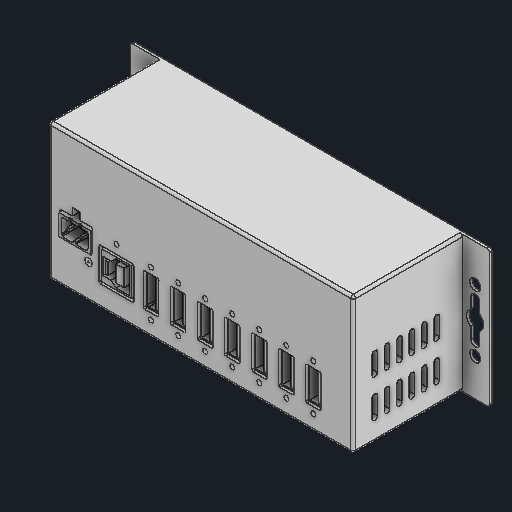
# Autodesk Inventor part: StarTech7PortUSB3Hub
Saved by Autodesk Inventor 2025.2 (Build 292293000, 293)
## iProperties
Created: 2025-10-31
Part Number: StarTech7PortUSB3Hub
Material: Generic
Document SubType Name: Modeling
Designer: valer
Density: 1 g/cm^3
Appearance: Default
Author: valer
Autodesk Inventor part; units mm, degrees
ref_plane "YZ Plane" through (0, 0, 0) normal (1, 0, 0) x (0, 1, 0)
ref_plane "XZ Plane" through (0, 0, 0) normal (0, 1, 0) x (-1, 0, 0)
ref_plane "XY Plane" through (0, 0, 0) normal (0, 0, 1) x (1, 0, 0)
sketch "Base" plane through (0, 0, 0) normal (0, 0, 1) x (1, 0, 0)
  line L0 (-72.5, -27.5) -> (72.5, -27.5)
  line L1 (72.5, -27.5) -> (72.5, 27.5)
  line L2 (72.5, 27.5) -> (-72.5, 27.5)
  line L3 (-72.5, 27.5) -> (-72.5, -27.5)
  line L4 (-72.5, -27.5) -> (72.5, 27.5) construction
  line L5 (72.5, -27.5) -> (-72.5, 27.5) construction
  line L6 (-66.75, 27.5) -> (-66.75, -27.5) construction
  line L7 (-101.5, 0) -> (101.5, 0) construction
  line L8 (0, -38.5) -> (0, 38.5) construction
  line L9 (66.75, 27.5) -> (66.75, -27.5) construction
  circle A0 centre (-66.75, 12.5) radius 2.25
  circle A1 centre (-66.75, -12.5) radius 2.25
  circle A2 centre (66.75, 12.5) radius 2.25
  circle A3 centre (66.75, -12.5) radius 2.25
  circle A4 centre (-66.75, 0) radius 3.5
  circle A5 centre (66.75, 0) radius 3.5
  circle A6 centre (-66.75, 7.5) radius 1.75
  circle A7 centre (-66.75, -7.5) radius 1.75
  line L10 (-68.5, 7.5) -> (-68.5, -7.5)
  line L11 (-65, 7.5) -> (-65, -7.5)
  circle A8 centre (66.75, 7.5) radius 1.75
  circle A9 centre (66.75, -7.5) radius 1.75
  line L12 (68.5, 7.5) -> (68.5, -7.5)
  line L13 (65, 7.5) -> (65, -7.5)
  line L14 (-70.25, 3.5) -> (-63.25, 3.5)
  line L15 (-63.25, 3.5) -> (-63.25, -3.5)
  line L16 (-63.25, -3.5) -> (-70.25, -3.5)
  line L17 (-70.25, -3.5) -> (-70.25, 3.5)
  point P0 (0, 0)
  point P1 (-65, -3.0311)
  point P2 (-68.5, -3.0311)
  point P3 (-68.5, 3.0311)
  point P4 (-65, 3.0311)
  point P5 (65, -3.0311)
  point P6 (65, 3.0311)
  point P7 (68.5, 3.0311)
  point P8 (68.5, -3.0311)
  dimension "d15" = 1
  dimension "d0" = 145
  dimension "d1" = 55
  dimension "d2" = 133.5
  dimension "d3" = 4.5
  dimension "d4" = 15
  dimension "d5" = 7
  dimension "d6" = 3.5
  dimension "d7" = 20
  dimension "d63" = 2.25
  constraints: 32 end point, 13 symmetric about line, 10 centre point, 8 point on circle, 8 tangent, 5 point on line, 4 parallel, 3 midpoint, 3 perpendicular, 2 horizontal, 7 other
  measures "d0" distance of L1.end L2.end
  measures "d1" distance of L0.end L1.end
  measures "d2" distance between parallel lines of L9 L6
  measures "d3" diameter of A0
  measures "d4" distance from line of L2 A0.centre
  measures "d5" diameter of A4
  measures "d6" diameter of A6
  measures "d7" distance of A1.centre A6.centre
  measures "d63" distance between parallel lines of L3 L17
extrude "BaseFeature" add sketch "Base" along normal blind 1 contours L3 L2 L1 L0 | L15 L16 L11 A4 | A4 L11 L14 L15 | A4 L17 L14 L10 | L10 L16 L17 A4
fillet "BaseFilletsFeature" radius 1 4 edges at (-72.5, -27.5, 0.5) (-72.5, 27.5, 0.5) (72.5, -27.5, 0.5) (72.5, 27.5, 0.5)
sketch "Sketch2" plane through (0, 0, 1) normal (0, 0, 1) x (1, 0, 0)
  line L0 (71.5, 27.5) -> (-71.5, 27.5) projected
  line L1 (-71.5, -27.5) -> (71.5, -27.5) projected
  line L2 (-61.5, 27.5) -> (61.5, 27.5)
  line L3 (61.5, 27.5) -> (61.5, -27.5)
  line L4 (61.5, -27.5) -> (-61.5, -27.5)
  line L5 (-61.5, -27.5) -> (-61.5, 27.5)
  line L6 (-72.5, 26.5) -> (-72.5, -26.5) projected
  line L7 (72.5, -26.5) -> (72.5, 26.5) projected
  point P0 (0, 0)
  point P1 (-61.5, -27.5)
  point P2 (61.5, 27.5)
  dimension "d11" = 11
  dimension "d12" = 11
  constraints: 8 end point, 2 parallel, 2 point on line, 1 horizontal, 1 perpendicular
  measures "d11" distance between parallel lines of L6 L5
  measures "d12" distance between parallel lines of L7 L3
extrude "BodyFeature" add sketch "Sketch2" along normal blind 44
fillet "BodyFilletsFeature" radius 1 4 edges at (-61.5, -27.5, 23) (-61.5, 27.5, 23) (61.5, -27.5, 23) (61.5, 27.5, 23)
sketch "Sketch3" plane through (0, 0, 45) normal (0, 0, 1) x (1, 0, 0)
  line L0 (-41.05, -1.85) -> (48.52, -1.85) construction
  line L1 (48.52, -1.85) -> (48.52, -22.35) construction
  line L2 (48.52, -22.35) -> (-41.05, -22.35) construction
  line L3 (-41.05, -22.35) -> (-41.05, -1.85) construction
  arc A0 (65, 3.0311) -> (65, -3.0311) centre (66.75, 0) ccw projected
  line L4 (48.52, -2.85) -> (-41.05, -2.85) construction
  line L5 (48.52, -12.1) -> (-41.05, -12.1) construction
  circle A1 centre (45.42, -2.85) radius 1
  line L6 (42.32, -5.35) -> (48.52, -5.35)
  line L7 (48.52, -5.35) -> (48.52, -18.85)
  line L8 (48.52, -18.85) -> (42.32, -18.85)
  line L9 (42.32, -18.85) -> (42.32, -5.35)
  line L10 (45.42, -2.85) -> (45.42, -12.1) construction
  circle A2 centre (45.42, -21.35) radius 1
  line L11 (61.5, -26.5) -> (61.5, 26.5) construction
  line L12 (31.4, -5.35) -> (37.6, -5.35)
  line L13 (31.4, -18.85) -> (31.4, -5.35)
  line L14 (37.6, -18.85) -> (31.4, -18.85)
  line L15 (37.6, -5.35) -> (37.6, -18.85)
  circle A3 centre (34.5, -2.85) radius 1
  circle A4 centre (34.5, -21.35) radius 1
  line L16 (20.48, -5.35) -> (26.68, -5.35)
  line L17 (20.48, -18.85) -> (20.48, -5.35)
  line L18 (26.68, -18.85) -> (20.48, -18.85)
  line L19 (26.68, -5.35) -> (26.68, -18.85)
  circle A5 centre (23.58, -2.85) radius 1
  circle A6 centre (23.58, -21.35) radius 1
  line L20 (9.56, -5.35) -> (15.76, -5.35)
  line L21 (9.56, -18.85) -> (9.56, -5.35)
  line L22 (15.76, -18.85) -> (9.56, -18.85)
  line L23 (15.76, -5.35) -> (15.76, -18.85)
  circle A7 centre (12.66, -2.85) radius 1
  circle A8 centre (12.66, -21.35) radius 1
  line L24 (-1.36, -5.35) -> (4.84, -5.35)
  line L25 (-1.36, -18.85) -> (-1.36, -5.35)
  line L26 (4.84, -18.85) -> (-1.36, -18.85)
  line L27 (4.84, -5.35) -> (4.84, -18.85)
  circle A9 centre (1.74, -2.85) radius 1
  circle A10 centre (1.74, -21.35) radius 1
  line L28 (-12.28, -5.35) -> (-6.08, -5.35)
  line L29 (-12.28, -18.85) -> (-12.28, -5.35)
  line L30 (-6.08, -18.85) -> (-12.28, -18.85)
  line L31 (-6.08, -5.35) -> (-6.08, -18.85)
  circle A11 centre (-9.18, -2.85) radius 1
  circle A12 centre (-9.18, -21.35) radius 1
  line L32 (-23.2, -5.35) -> (-17, -5.35)
  line L33 (-23.2, -18.85) -> (-23.2, -5.35)
  line L34 (-17, -18.85) -> (-23.2, -18.85)
  line L35 (-17, -5.35) -> (-17, -18.85)
  circle A13 centre (-20.1, -2.85) radius 1
  circle A14 centre (-20.1, -21.35) radius 1
  line L36 (-27.05, -5.35) -> (-41.05, -5.35)
  line L37 (-41.05, -5.35) -> (-41.05, -18.85)
  line L38 (-41.05, -18.85) -> (-27.05, -18.85)
  line L39 (-27.05, -18.85) -> (-27.05, -5.35)
  line L40 (-34.05, -2.85) -> (-34.05, -22.35) construction
  line L41 (-56.85, -0.85) -> (-43.85, -0.85)
  line L42 (-43.85, -0.85) -> (-43.85, -10.25)
  line L43 (-43.85, -10.25) -> (-56.85, -10.25)
  line L44 (-56.85, -10.25) -> (-56.85, -0.85)
  line L45 (-61.5, 26.5) -> (-61.5, -26.5) construction
  circle A15 centre (-34.05, -1.85) radius 1
  circle A16 centre (-34.05, -22.35) radius 1
  circle A17 centre (-45.35, -13.6) radius 1.5
  line L46 (-43.85, -10.25) -> (-43.85, -13.6) construction
  line L47 (-41.05, -12.1) -> (-45.35, -12.1) construction
  line L48 (-51.85, -0.85) -> (-48.85, -0.85)
  line L49 (-48.85, -0.85) -> (-48.85, 2.15)
  line L50 (-48.85, 2.15) -> (-51.85, 2.15)
  line L51 (-51.85, 2.15) -> (-51.85, -0.85)
  line L52 (-50.35, -10.25) -> (-50.35, -0.85) construction
  point P0 (0, 0)
  point P1 (42.32, -12.1)
  point P2 (45.42, -5.35)
  point P3 (34.5, -5.35)
  point P4 (31.4, -12.1)
  point P5 (23.58, -5.35)
  point P6 (20.48, -12.1)
  point P7 (12.66, -5.35)
  point P8 (9.56, -12.1)
  point P9 (1.74, -5.35)
  point P10 (-1.36, -12.1)
  point P11 (-9.18, -5.35)
  point P12 (-12.28, -12.1)
  point P13 (-20.1, -5.35)
  point P14 (-23.2, -12.1)
  point P15 (-34.05, -5.35)
  point P16 (-27.05, -12.1)
  point P17 (-50.35, -0.85)
  dimension "d16" = 12.1
  dimension "d17" = 2
  dimension "d18" = 13.5
  dimension "d19" = 6.2
  dimension "d20" = 18.5
  dimension "d21" = 12.98
  dimension "d24" = 10.92
  dimension "d29" = 14
  dimension "d30" = 13.95
  dimension "d31" = 16.3
  dimension "d32" = 9.4
  dimension "d33" = 11.15
  dimension "d34" = 1
  dimension "d35" = 13
  dimension "d36" = 3
  dimension "d64" = 3
  constraints: 102 end point, 17 centre point, 13 point on line, 10 midpoint, 10 parallel, 9 perpendicular, 6 horizontal, 4 collinear, 3 tangent, 2 equal length, 2 equal radius, 2 point on circle, 1 coincident, 1 symmetric about line, 85 other
  measures "d16" vertical distance of A0.centre L5.start
  measures "d17" diameter of A1
  measures "d18" distance of L6.end L7.end
  measures "d19" distance between parallel lines of L9 L7
  measures "d20" distance from line of A2.centre L4
  measures "d21" distance between parallel lines of L11 L1
  measures "d24" distance of L6.start L12.start
  measures "d29" distance of L37.end L38.end
  measures "d30" distance from line of A14.centre L40
  measures "d31" distance from line of L52.start L40
  measures "d32" distance of L41.end L42.end
  measures "d33" distance from line of L45 L52.start
  measures "d34" distance between parallel lines of L0 L41
  measures "d35" distance of L42.end L43.end
  measures "d36" diameter of A17
  measures "d64" distance of L49.end L50.end
extrude "PortsFeature" cut sketch "Sketch3" against normal blind 6 contours A1 | L6 L7 L8 L9 | A2 | L12 L15 L14 L13 | A3 | A4 | L16 L19 L18 L17 | A5 | A6 | L20 L23 L22 L21 | A7 | A8 | L24 L27 L26 L25 | A9 | A10 | L28 L31 L30 L29 | A11 | A12 | L32 L35 L34 L33 | A13 | A14 | L39 L38 L37 L36 | L41 L42 L43 L44 | L51 L50 L49 L41 | A15 | A17
fillet "PortFilletsFeature" radius 0.5 36 edges at (48.52, -5.35, 42) (42.32, -5.35, 42) (42.32, -18.85, 42) (48.52, -18.85, 42) (37.6, -5.35, 42) (31.4, -5.35, 42) (31.4, -18.85, 42) (37.6, -18.85, 42) (26.68, -5.35, 42) (20.48, -5.35, 42) (20.48, -18.85, 42) (26.68, -18.85, 42) (15.76, -5.35, 42) (9.56, -5.35, 42) (9.56, -18.85, 42) (15.76, -18.85, 42) (4.84, -5.35, 42) (-1.36, -5.35, 42) (-1.36, -18.85, 42) (4.84, -18.85, 42) (-6.08, -5.35, 42) (-12.28, -5.35, 42) (-12.28, -18.85, 42) (-6.08, -18.85, 42) (-17, -5.35, 42) (-23.2, -5.35, 42) (-23.2, -18.85, 42) (-17, -18.85, 42) (-27.05, -5.35, 42) (-41.05, -5.35, 42) (-41.05, -18.85, 42) (-27.05, -18.85, 42) (-43.85, -0.85, 42) (-56.85, -0.85, 42) (-56.85, -10.25, 42) (-43.85, -10.25, 42)
fillet "OutsideFilletsFeature" radius 1 8 edges at (-61.2071, 27.2071, 45) (-61.5, 0, 45) (-61.2071, -27.2071, 45) (0, -27.5, 45) (61.2071, -27.2071, 45) (61.5, 0, 45) (61.2071, 27.2071, 45) (0, 27.5, 45)
sketch "Vents" plane through (61.5, -26.5, 1) normal (1, 0, 0) x (0, 0, -1)
  line L0 (-44, 7.65) -> (-38, 7.65) construction
  line L1 (-35.35, 7.65) -> (0, 7.65) construction
  line L2 (0, 7.65) -> (0, 15.65) construction
  line L3 (0, 15.65) -> (-35.35, 15.65) construction
  line L4 (-35.35, 15.65) -> (-35.35, 7.65) construction
  line L5 (-43, -1) -> (0, -1) projected
  line L6 (-44, 53) -> (-44, 0) projected
  line L7 (-35.35, 22.85) -> (-35.35, 14.85) construction
  line L8 (-35.35, 14.85) -> (0, 14.85) construction
  line L9 (0, 22.85) -> (-35.35, 22.85) construction
  line L10 (0, 14.85) -> (0, 22.85) construction
  line L11 (-35.35, 30.05) -> (-35.35, 22.05) construction
  line L12 (-35.35, 22.05) -> (0, 22.05) construction
  line L13 (0, 30.05) -> (-35.35, 30.05) construction
  line L14 (0, 22.05) -> (0, 30.05) construction
  line L15 (-35.35, 7.65) -> (-35.35, 14.85) construction
  line L16 (-34.25, 7.65) -> (-34.25, 14.85)
  line L17 (-36.45, 14.85) -> (-36.45, 7.65)
  arc A0 (-36.45, 7.65) -> (-34.25, 7.65) centre (-35.35, 7.65) ccw
  arc A1 (-34.25, 14.85) -> (-36.45, 14.85) centre (-35.35, 14.85) ccw
  line L18 (0, 0) -> (0, 53) projected
  line L19 (-35.35, 18.85) -> (0, 18.85) construction
  line L20 (-34.25, 30.05) -> (-34.25, 22.85)
  line L21 (-36.45, 22.85) -> (-36.45, 30.05)
  arc A2 (-34.25, 30.05) -> (-36.45, 30.05) centre (-35.35, 30.05) ccw
  arc A3 (-36.45, 22.85) -> (-34.25, 22.85) centre (-35.35, 22.85) ccw
  arc A4 (-31.45, 7.65) -> (-29.25, 7.65) centre (-30.35, 7.65) ccw
  line L22 (-31.45, 14.85) -> (-31.45, 7.65)
  line L23 (-29.25, 7.65) -> (-29.25, 14.85)
  arc A5 (-29.25, 14.85) -> (-31.45, 14.85) centre (-30.35, 14.85) ccw
  arc A6 (-31.45, 22.85) -> (-29.25, 22.85) centre (-30.35, 22.85) ccw
  line L24 (-31.45, 22.85) -> (-31.45, 30.05)
  line L25 (-29.25, 30.05) -> (-29.25, 22.85)
  arc A7 (-29.25, 30.05) -> (-31.45, 30.05) centre (-30.35, 30.05) ccw
  arc A8 (-26.45, 7.65) -> (-24.25, 7.65) centre (-25.35, 7.65) ccw
  line L26 (-26.45, 14.85) -> (-26.45, 7.65)
  line L27 (-24.25, 7.65) -> (-24.25, 14.85)
  arc A9 (-24.25, 14.85) -> (-26.45, 14.85) centre (-25.35, 14.85) ccw
  arc A10 (-26.45, 22.85) -> (-24.25, 22.85) centre (-25.35, 22.85) ccw
  line L28 (-26.45, 22.85) -> (-26.45, 30.05)
  line L29 (-24.25, 30.05) -> (-24.25, 22.85)
  arc A11 (-24.25, 30.05) -> (-26.45, 30.05) centre (-25.35, 30.05) ccw
  arc A12 (-21.45, 7.65) -> (-19.25, 7.65) centre (-20.35, 7.65) ccw
  line L30 (-21.45, 14.85) -> (-21.45, 7.65)
  line L31 (-19.25, 7.65) -> (-19.25, 14.85)
  arc A13 (-19.25, 14.85) -> (-21.45, 14.85) centre (-20.35, 14.85) ccw
  arc A14 (-21.45, 22.85) -> (-19.25, 22.85) centre (-20.35, 22.85) ccw
  line L32 (-21.45, 22.85) -> (-21.45, 30.05)
  line L33 (-19.25, 30.05) -> (-19.25, 22.85)
  arc A15 (-19.25, 30.05) -> (-21.45, 30.05) centre (-20.35, 30.05) ccw
  arc A16 (-16.45, 7.65) -> (-14.25, 7.65) centre (-15.35, 7.65) ccw
  line L34 (-16.45, 14.85) -> (-16.45, 7.65)
  line L35 (-14.25, 7.65) -> (-14.25, 14.85)
  arc A17 (-14.25, 14.85) -> (-16.45, 14.85) centre (-15.35, 14.85) ccw
  arc A18 (-16.45, 22.85) -> (-14.25, 22.85) centre (-15.35, 22.85) ccw
  line L36 (-16.45, 22.85) -> (-16.45, 30.05)
  line L37 (-14.25, 30.05) -> (-14.25, 22.85)
  arc A19 (-14.25, 30.05) -> (-16.45, 30.05) centre (-15.35, 30.05) ccw
  arc A20 (-11.45, 7.65) -> (-9.25, 7.65) centre (-10.35, 7.65) ccw
  line L38 (-11.45, 14.85) -> (-11.45, 7.65)
  line L39 (-9.25, 7.65) -> (-9.25, 14.85)
  arc A21 (-9.25, 14.85) -> (-11.45, 14.85) centre (-10.35, 14.85) ccw
  arc A22 (-11.45, 22.85) -> (-9.25, 22.85) centre (-10.35, 22.85) ccw
  line L40 (-11.45, 22.85) -> (-11.45, 30.05)
  line L41 (-9.25, 30.05) -> (-9.25, 22.85)
  arc A23 (-9.25, 30.05) -> (-11.45, 30.05) centre (-10.35, 30.05) ccw
  point P0 (1, 26.5)
  point P1 (-35.35, 11.25)
  dimension "d41" = 8.65
  dimension "d42" = 8.65
  dimension "d46" = 7.2
  dimension "d51" = 1.1
  dimension "d54" = 5
  dimension "d59" = 7.2
  dimension "d60" = 8
  constraints: 78 end point, 48 point on circle, 24 centre point, 5 symmetric about line, 4 tangent, 3 collinear, 3 parallel, 2 horizontal, 2 midpoint, 2 perpendicular, 2 point on line, 1 vertical, 117 other
  measures "d41" distance between parallel lines of L5 L0
  measures "d42" distance between parallel lines of L6 L4
  measures "d46" distance of L3.end L7.start
  measures "d51" radius of A1
  measures "d54" distance of L1.start A4.centre
  measures "d59" distance between parallel lines of L0 L8
  measures "d60" distance between parallel lines of L9 L8
extrude "VentsFeature" cut sketch "Vents" against normal blind 20
sketch "Sketch5" plane through (-45.35, -13.6, 39) normal (0, 0, 1) x (1, 0, 0)
  circle A0 centre (0, 0) radius 1.5 projected
  circle A1 centre (0, 0) radius 1.3
  point P0 (45.35, 13.6)
  dimension "d65" = 0.2
  constraints: 1 centre point
  measures "d65" radial gap between concentric circles of A0 A1
extrude "Extrusion5" add sketch "Sketch5" along normal blind 6 contours A1
fillet "Fillet5" radius 1 1 edges at (-46.65, -13.6, 45)
sketch "Sketch6" plane through (0, 0, 39) normal (0, 0, 1) x (1, 0, 0)
  line L0 (-56.85, -1.85) -> (-43.85, -1.85)
  line L1 (-43.85, -1.85) -> (-43.85, -10.25)
  line L2 (-43.85, -10.25) -> (-56.85, -10.25)
  line L3 (-56.85, -10.25) -> (-56.85, -1.85)
  line L4 (-48.85, -0.85) -> (-44.35, -0.85) projected
  line L5 (-43.85, -1.35) -> (-43.85, -9.75) projected
  line L6 (-44.35, -10.25) -> (-56.35, -10.25) projected
  line L7 (-56.85, -9.75) -> (-56.85, -1.35) projected
  line L8 (-44.85, -2.85) -> (-55.85, -2.85)
  line L9 (-55.85, -2.85) -> (-55.85, -9.25)
  line L10 (-55.85, -9.25) -> (-44.85, -9.25) construction
  line L11 (-44.85, -9.25) -> (-44.85, -2.85)
  line L12 (-50.35, -2.85) -> (-50.35, -9.25) construction
  arc A0 (-55.85, -9.25) -> (-50.35, -9.25) centre (-53.1, 0.3644) ccw
  arc A1 (-50.35, -9.25) -> (-44.85, -9.25) centre (-47.6, 0.3644) ccw
  line L13 (-55.85, -2.85) -> (-50.35, -9.25) construction
  line L14 (-50.35, -9.25) -> (-44.85, -2.85) construction
  line L15 (-53.6, -5.55) -> (-52.6, -5.55)
  line L16 (-52.6, -5.55) -> (-52.6, -6.55)
  line L17 (-52.6, -6.55) -> (-53.6, -6.55)
  line L18 (-53.6, -6.55) -> (-53.6, -5.55)
  line L19 (-53.6, -5.55) -> (-52.6, -6.55) construction
  line L20 (-52.6, -5.55) -> (-53.6, -6.55) construction
  line L21 (-47.1, -5.55) -> (-48.1, -5.55)
  line L22 (-48.1, -5.55) -> (-48.1, -6.55)
  line L23 (-48.1, -6.55) -> (-47.1, -6.55)
  line L24 (-47.1, -6.55) -> (-47.1, -5.55)
  point P0 (0, 0)
  point P1 (-53.1, -6.05)
  dimension "d69" = 1
  dimension "d70" = 1
  dimension "d71" = 10
  dimension "d72" = 1
  constraints: 42 end point, 6 parallel, 5 midpoint, 4 perpendicular, 4 point on circle, 4 symmetric about line, 3 collinear, 2 centre point, 2 horizontal, 1 equal radius, 3 other
  measures "d69" distance between parallel lines of L0 L4
  measures "d70" distance between parallel lines of L0 L8
  measures "d71" radius of A0
  measures "d72" distance of L15.end L16.end
extrude "Extrusion6" add sketch "Sketch6" along normal blind 6.5
sketch "Sketch7" plane through (0, 0, 45.5) normal (0, 0, 1) x (1, 0, 0)
  line L0 (-43.85, -1.85) -> (-56.85, -1.85) projected
  line L1 (-44.85, -2.85) -> (-44.85, -9.25) projected
  arc A0 (-50.35, -9.25) -> (-44.85, -9.25) centre (-47.6, 0.3644) ccw projected
  arc A1 (-55.85, -9.25) -> (-50.35, -9.25) centre (-53.1, 0.3644) ccw projected
  line L2 (-55.85, -9.25) -> (-55.85, -2.85) projected
  line L3 (-55.85, -2.85) -> (-44.85, -2.85) projected
  line L4 (-56.35, -9.75) -> (-55.35, -9.75)
  line L5 (-55.35, -9.75) -> (-55.35, -8.75)
  line L6 (-55.35, -8.75) -> (-56.35, -8.75)
  line L7 (-56.35, -8.75) -> (-56.35, -9.75)
  line L8 (-56.35, -9.75) -> (-55.35, -8.75) construction
  line L9 (-55.35, -9.75) -> (-56.35, -8.75) construction
  line L10 (-55.85, -2.85) -> (-55.85, -9.25) projected
  line L11 (-55.85, -6.05) -> (-44.85, -6.05) construction
  line L12 (-50.35, -2.85) -> (-50.35, -9.25) construction
  line L13 (-44.35, -9.75) -> (-45.35, -9.75)
  line L14 (-45.35, -9.75) -> (-45.35, -8.75)
  line L15 (-45.35, -8.75) -> (-44.35, -8.75)
  line L16 (-44.35, -8.75) -> (-44.35, -9.75)
  line L17 (-56.35, -2.35) -> (-55.35, -2.35)
  line L18 (-55.35, -2.35) -> (-55.35, -3.35)
  line L19 (-55.35, -3.35) -> (-56.35, -3.35)
  line L20 (-56.35, -3.35) -> (-56.35, -2.35)
  line L21 (-45.35, -2.35) -> (-45.35, -3.35)
  line L22 (-45.35, -3.35) -> (-44.35, -3.35)
  line L23 (-44.35, -3.35) -> (-44.35, -2.35)
  line L24 (-44.35, -2.35) -> (-45.35, -2.35)
  line L25 (-50.85, -9.75) -> (-49.85, -9.75)
  line L26 (-49.85, -9.75) -> (-49.85, -8.75)
  line L27 (-49.85, -8.75) -> (-50.85, -8.75)
  line L28 (-50.85, -8.75) -> (-50.85, -9.75)
  line L29 (-50.85, -9.75) -> (-49.85, -8.75) construction
  line L30 (-49.85, -9.75) -> (-50.85, -8.75) construction
  line L31 (-55.85, -8.75) -> (-55.35, -8.75)
  line L32 (-55.35, -8.75) -> (-55.35, -9.3791)
  line L33 (-56.85, -1.85) -> (-56.85, -10.25) projected
  line L34 (-56.85, -10.25) -> (-43.85, -10.25) projected
  line L35 (-43.85, -10.25) -> (-43.85, -1.85) projected
  point P0 (0, 0)
  point P1 (-50.85, -9.3791)
  point P2 (-49.85, -9.3791)
  point P3 (-44.85, -8.75)
  point P4 (-45.35, -9.3791)
  dimension "d75" = 1
  constraints: 56 end point, 12 symmetric about line, 8 midpoint, 4 parallel, 3 equal length, 2 horizontal, 2 perpendicular, 2 point on line, 1 collinear, 1 point on circle, 1 vertical
  measures "d75" distance of L6.end L5.end
extrude "Extrusion7" add sketch "Sketch7" against normal up to surface (6.5 mm away) contours L3 L21 L24 L23 L22 L1 | L1 L22 L21 L3 | L1 A0 L14 L15 | L18 L19 L2 L3 | L3 L2 L19 L20 L17 L18 | A0 A1 L28 L27 L26 | L6 L5 A1 L2
sketch "Sketch8" plane through (0, 0, 45.5) normal (0, 0, 1) x (1, 0, 0)
  line L0 (-50.85, -8.75) -> (-49.85, -8.75) construction
  line L1 (-50.35, -8.75) -> (-50.35, -1.85) construction
  line L2 (-43.85, -1.85) -> (-56.85, -1.85) construction
  line L3 (-55.35, -2.85) -> (-45.35, -2.85) projected
  line L4 (-52.85, -1.85) -> (-51.85, -1.85)
  line L5 (-51.85, -1.85) -> (-51.85, -2.85)
  line L6 (-51.85, -2.85) -> (-52.85, -2.85)
  line L7 (-52.85, -2.85) -> (-52.85, -1.85)
  line L8 (-51.85, -0.85) -> (-51.85, 2.15) projected
  line L9 (-47.85, -1.85) -> (-48.85, -1.85)
  line L10 (-48.85, -1.85) -> (-48.85, -2.85)
  line L11 (-48.85, -2.85) -> (-47.85, -2.85)
  line L12 (-47.85, -2.85) -> (-47.85, -1.85)
  point P0 (0, 0)
  dimension "d78" = 1
  constraints: 18 end point, 4 symmetric about line, 2 midpoint, 2 parallel, 2 point on line, 1 collinear, 1 horizontal, 1 perpendicular
  measures "d78" distance between parallel lines of L5 L7
extrude "Extrusion8" cut sketch "Sketch8" against normal blind 0.5
sketch "Sketch9" plane through (0, 0, 39) normal (0, 0, 1) x (1, 0, 0)
  line L0 (-28.05, -6.35) -> (-40.05, -6.35)
  line L1 (-40.05, -6.35) -> (-40.05, -17.85)
  line L2 (-40.05, -17.85) -> (-28.05, -17.85)
  line L3 (-28.05, -17.85) -> (-28.05, -6.35)
  line L4 (-40.05, -12.1) -> (-28.05, -12.1) construction
  line L5 (-39.55, -12.1) -> (-39.55, -8.7282)
  line L6 (-39.55, -8.7282) -> (-36.25, -8.7282)
  line L7 (-36.25, -8.7282) -> (-34.25, -7.05)
  line L8 (-34.25, -7.05) -> (-28.75, -7.05)
  line L9 (-28.75, -7.05) -> (-28.75, -12.1)
  line L10 (-40.55, -5.35) -> (-27.55, -5.35) projected
  line L11 (-27.05, -5.85) -> (-27.05, -18.35) projected
  line L12 (-41.05, -18.35) -> (-41.05, -5.85) projected
  line L13 (-27.55, -18.85) -> (-40.55, -18.85) projected
  line L14 (-39.55, -12.1) -> (-39.55, -15.4718)
  line L15 (-39.55, -15.4718) -> (-36.25, -15.4718)
  line L16 (-36.25, -15.4718) -> (-34.25, -17.15)
  line L17 (-34.25, -17.15) -> (-28.75, -17.15)
  line L18 (-28.75, -17.15) -> (-28.75, -12.1)
  line L19 (-34.25, -15.45) -> (-31.05, -15.45)
  line L20 (-31.05, -15.45) -> (-31.05, -8.75)
  line L21 (-31.05, -8.75) -> (-34.25, -8.75)
  line L22 (-34.25, -8.75) -> (-34.25, -15.45)
  line L23 (-34.25, -15.45) -> (-31.05, -8.75) construction
  line L24 (-31.05, -15.45) -> (-34.25, -8.75) construction
  line L25 (-34.25, -7.05) -> (-34.25, -8.75) construction
  line L26 (-38.55, -14.4718) -> (-38.55, -9.7282)
  line L27 (-38.55, -9.7282) -> (-37.55, -9.7282)
  line L28 (-37.55, -9.7282) -> (-37.55, -14.4718)
  line L29 (-37.55, -14.4718) -> (-38.55, -14.4718)
  line L30 (-38.55, -14.4718) -> (-37.55, -9.7282) construction
  line L31 (-38.55, -9.7282) -> (-37.55, -14.4718) construction
  point P0 (0, 0)
  point P1 (-32.65, -12.1)
  point P2 (-38.05, -12.1)
  dimension "d81" = 1
  dimension "d82" = 1
  dimension "d83" = 1
  dimension "d84" = 0.5
  dimension "d85" = 0.7
  dimension "d86" = 0.7
  dimension "d87" = 140
  dimension "d88" = 3.3
  dimension "d89" = 5.5
  dimension "d90" = 1
  dimension "d91" = 2.3
  dimension "d92" = 1.7
  dimension "d95" = 1
  dimension "d96" = 1
  dimension "d97" = 1
  constraints: 56 end point, 7 parallel, 7 perpendicular, 6 midpoint, 4 point on line, 4 symmetric about line, 2 horizontal, 1 vertical
  measures "d81" distance between parallel lines of L10 L0
  measures "d82" distance between parallel lines of L11 L3
  measures "d83" distance between parallel lines of L12 L1
  measures "d84" distance between parallel lines of L1 L5
  measures "d85" distance between parallel lines of L0 L8
  measures "d86" distance between parallel lines of L3 L9
  measures "d87" angle of L6 L7
  measures "d88" distance of L5.end L6.end
  measures "d89" distance of L7.end L8.end
  measures "d90" distance between parallel lines of L13 L2
  measures "d91" distance between parallel lines of L9 L20
  measures "d92" distance between parallel lines of L8 L21
  measures "d95" distance between parallel lines of L6 L27
  measures "d96" distance between parallel lines of L5 L26
  measures "d97" distance of L26.end L27.end
extrude "Extrusion9" add sketch "Sketch9" along normal up to surface (6 mm away)
sketch "Sketch10" plane through (0, 0, 39) normal (0, 0, 1) x (1, 0, 0)
  line L0 (-23.2, -18.35) -> (-23.2, -5.85) construction
  line L1 (-23.2, -12.1) -> (-17, -12.1) construction
  line L2 (-17, -5.85) -> (-17, -18.35) construction
  line L3 (-23.0536, -12.1) -> (-23.0536, -5.4964)
  line L4 (-23.0536, -5.4964) -> (-17.1464, -5.4964)
  line L5 (-17.1464, -5.4964) -> (-17.1464, -12.1)
  arc A0 (-22.7, -5.35) -> (-23.2, -5.85) centre (-22.7, -5.85) ccw projected
  arc A1 (-17, -5.85) -> (-17.5, -5.35) centre (-17.5, -5.85) ccw projected
  line L6 (-17.6464, -12.1) -> (-17.6464, -5.9964)
  line L7 (-17.6464, -5.9964) -> (-22.5536, -5.9964)
  line L8 (-22.5536, -5.9964) -> (-22.5536, -12.1)
  line L9 (-23.0536, -12.1) -> (-23.0536, -18.7036)
  line L10 (-23.0536, -18.7036) -> (-17.1464, -18.7036)
  line L11 (-17.1464, -18.7036) -> (-17.1464, -12.1)
  line L12 (-17.6464, -12.1) -> (-17.6464, -18.2036)
  line L13 (-17.6464, -18.2036) -> (-22.5536, -18.2036)
  line L14 (-22.5536, -18.2036) -> (-22.5536, -12.1)
  point P0 (0, 0)
  dimension "d101" = 0.5
  constraints: 26 end point, 4 symmetric about line, 3 perpendicular, 2 midpoint, 2 point on circle, 2 point on line, 1 vertical, 2 other
  measures "d101" distance between parallel lines of L4 L7
extrude "Extrusion10" add sketch "Sketch10" along normal blind 5 separate body
chamfer "Chamfer2" distance 0.5 angle 45 8 edges at (-23.0536, -5.4964, 41.5) (-17.1464, -5.4964, 41.5) (-23.0536, -18.7036, 41.5) (-17.1464, -18.7036, 41.5) (-22.5536, -5.9964, 41.5) (-17.6464, -5.9964, 41.5) (-22.5536, -18.2036, 41.5) (-17.6464, -18.2036, 41.5)
sketch "Sketch11" plane through (0, 0, 39) normal (0, 0, 1) x (1, 0, 0)
  line L0 (-18.1464, -6.4964) -> (-19.1464, -6.4964)
  line L1 (-19.1464, -6.4964) -> (-19.1464, -17.7036)
  line L2 (-19.1464, -17.7036) -> (-18.1464, -17.7036)
  line L3 (-18.1464, -17.7036) -> (-18.1464, -6.4964)
  line L4 (-22.0536, -5.9964) -> (-18.1464, -5.9964) projected
  line L5 (-18.1464, -6.4964) -> (-18.1464, -5.9964) construction
  line L6 (-22.0536, -5.9964) -> (-18.1464, -5.9964) projected
  line L7 (-17.6464, -6.4964) -> (-17.6464, -17.7036) projected
  line L8 (-18.1464, -6.4964) -> (-17.6464, -6.4964) construction
  line L9 (-18.1464, -18.2036) -> (-17.6464, -17.7036) projected
  line L10 (-18.1464, -18.2036) -> (-18.1464, -17.7036) construction
  line L11 (-18.1464, -17.7036) -> (-17.6464, -17.7036) construction
  point P0 (0, 0)
  dimension "d107" = 1
  constraints: 16 end point, 4 perpendicular, 2 parallel, 1 horizontal, 1 vertical
  measures "d107" distance between parallel lines of L3 L1
extrude "Extrusion11" add sketch "Sketch11" along normal blind 5 bodies 2
pattern_linear "Rectangular Pattern1" count 7 spacing 10.92 along (1, 0, 0) of "Extrusion10", "Extrusion11" bodies 2
combine bodies "Combine1" operation type add bodies to combine 2 1
equation "\"d42\" = d41"
body "Solid2"
